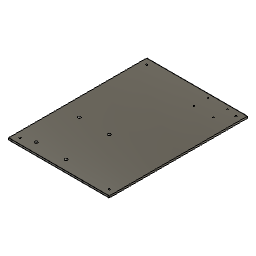
5780 Smaller Board v1 (Autodesk Fusion 360 design; units mm, degrees)
Autodesk Fusion 360 part; units mm, degrees
sketch "Sketch1" plane through (0, 0, 0) normal (0, 0, 1) x (1, 0, 0)
  line L0 (-65, 130) -> (110, 130)
  line L1 (110, 130) -> (110, -110)
  line L2 (110, -110) -> (-65, -110)
  line L3 (-65, -110) -> (-65, 130)
  dimension "d1" = 175
  dimension "d2" = 240
  constraint horizontal L0
  constraint vertical L1
  constraint horizontal L2
  constraint vertical L3
  measures "d1" distance of L1.end L2.end
  measures "d2" distance of L0.start L2.end
extrude "Extrude1" add sketch "Sketch1" along normal blind 3
sketch "Sketch2" plane through (0, 0, 3) normal (0, 0, 1) x (-1, 0, 0)
  line L0 (65, 110) -> (-110, 110)
  line L1 (-110, 110) -> (-110, -130)
  line L2 (-110, -130) -> (65, -130)
  line L3 (65, -130) -> (65, 110)
  circle A0 centre (34.5, 92.5) radius 2.5
  line L4 (60, 5.0001) -> (-105, 5)
  line L5 (12.025, 12.961) -> (3.6107, 13.032) construction
  line L6 (3.6107, 13.032) -> (3.5857, 10.071) construction
  line L7 (3.5857, 10.071) -> (12, 10) construction
  line L8 (12, 10) -> (12.025, 12.961) construction
  line L9 (-105, 5) -> (-105, 105.0001)
  line L10 (-105, 105.0001) -> (60, 105.0001)
  line L11 (12, 100) -> (-4.2428, 100.0343) construction
  line L12 (-4.2428, 100.0343) -> (-4.2609, 91.4763) construction
  line L13 (-4.2609, 91.4763) -> (11.9819, 91.4419) construction
  line L14 (11.9819, 91.4419) -> (12, 100) construction
  line L15 (60, 105.0001) -> (60, 5.0001)
  circle A1 centre (-17.5, 17.5) radius 2.5
  circle A2 centre (-17.5, 92.5) radius 2.5
  circle A3 centre (34.5, 17.5) radius 2.5
  line L16 (-46.15, -125) -> (-84, -125)
  line L17 (-84, -125) -> (-84, -97)
  line L18 (-84, -97) -> (-46.15, -97)
  line L19 (-46.15, -97) -> (-46.15, -125)
  circle A4 centre (-47.975, -123.15) radius 1
  circle A5 centre (-82.175, -123.15) radius 1
  circle A6 centre (-47.975, -98.85) radius 1
  circle A7 centre (-82.175, -98.85) radius 1
  dimension "d33" = 10
  dimension "d34" = 10
  dimension "d7" = 100
  dimension "d8" = 165
  dimension "d9" = 5
  dimension "d10" = 5
  dimension "d11" = 5
  dimension "d12" = 5
  dimension "d13" = 52
  dimension "d14" = 75
  dimension "d15" = 52
  dimension "d16" = 75
  dimension "d17" = 25.5
  dimension "d18" = 25.5
  dimension "d19" = 12.5
  dimension "d20" = 87.5
  dimension "d21" = 12.5
  dimension "d22" = 5
  dimension "d23" = 48
  dimension "d24" = 5
  dimension "d25" = 48
  dimension "d26" = 12.5
  dimension "d27" = 87.5
  dimension "d28" = 5
  dimension "d29" = 5
  dimension "d76" = 37.85
  dimension "d77" = 28
  dimension "d78" = 2
  dimension "d79" = 2
  dimension "d80" = 2
  dimension "d81" = 2
  dimension "d82" = 34.2
  dimension "d83" = 24.3
  dimension "d84" = 34.2
  dimension "d85" = 24.3
  dimension "d86" = 1.825
  dimension "d87" = 1.825
  dimension "d88" = 1.825
  dimension "d89" = 1.825
  dimension "d90" = 1.85
  dimension "d91" = 1.85
  dimension "d92" = 1.85
  dimension "d93" = 1.85
  dimension "d94" = 26
  dimension "d95" = 5
  constraint horizontal L16
  constraint vertical L17
  constraint horizontal L18
  constraint vertical L19
  measures "d7" distance of L4.start L10.end
  measures "d8" distance of L4.start L4.end
  measures "d9" diameter of A3
  measures "d10" diameter of A0
  measures "d11" diameter of A1
  measures "d12" diameter of A2
  measures "d13" distance of A3.centre A1.centre
  measures "d14" distance of A3.centre A0.centre
  measures "d15" distance of A0.centre A2.centre
  measures "d16" distance of A1.centre A2.centre
  measures "d17" distance of A3.centre L15
  measures "d18" distance of A0.centre L15
  measures "d19" distance of A3.centre L4
  measures "d20" distance of A1.centre L9
  measures "d21" distance of A1.centre L4
  measures "d26" distance of A2.centre L10
  measures "d27" distance of A2.centre L9
  measures "d28" distance of L3 L15
  measures "d29" distance of L0 L10
  measures "d76" distance of L16.start L16.end
  measures "d77" distance of L16.start L18.end
  measures "d78" diameter of A4
  measures "d79" diameter of A5
  measures "d80" diameter of A6
  measures "d81" diameter of A7
  measures "d82" distance of A4.centre A5.centre
  measures "d83" distance of A4.centre A6.centre
  measures "d84" horizontal distance of A6.centre A7.centre
  measures "d85" distance of A5.centre A7.centre
  measures "d86" distance of L17 A5.centre
  measures "d87" distance of L17 A7.centre
  measures "d88" distance of L19 A6.centre
  measures "d89" distance of L19 A4.centre
  measures "d90" distance of L16 A4.centre
  measures "d91" distance of L16 A5.centre
  measures "d92" distance of L18 A6.centre
  measures "d93" distance of L18 A7.centre
  measures "d94" distance of L1 L17
  measures "d95" distance of L2 L16
extrude "Extrude2" cut sketch "Sketch2" against normal blind 3 contours A0 | A1 | A2 | A3 | A4 | A5 | A6 | A7
sketch "Sketch3" plane through (0, 0, 3) normal (0, 0, 1) x (-1, 0, 0)
  circle A0 centre (-47.975, -123.15) radius 1
  circle A1 centre (-17.5, 92.5) radius 2.5
  circle A2 centre (34.5, 17.5) radius 2.5
  circle A3 centre (-82.175, -123.15) radius 1
  circle A4 centre (-47.975, -98.85) radius 1
  circle A5 centre (34.5, 92.5) radius 2.5
  circle A6 centre (-17.5, 17.5) radius 2.5
  circle A7 centre (-82.175, -98.85) radius 1
  line L0 (65, 110) -> (-110, 110)
  line L1 (-110, 110) -> (-110, -130)
  line L2 (-110, -130) -> (65, -130)
  line L3 (65, -130) -> (65, 110)
  circle A8 centre (55, -120) radius 1.5
  circle A9 centre (-100, -120) radius 1.5
  circle A10 centre (-100, 100) radius 1.5
  circle A11 centre (55, 100) radius 1.5
  dimension "d98" = 3
  dimension "d99" = 10
  dimension "d100" = 10
  dimension "d101" = 3
  dimension "d102" = 10
  dimension "d103" = 10
  dimension "d104" = 3
  dimension "d105" = 10
  dimension "d106" = 10
  dimension "d107" = 3
  dimension "d108" = 10
  dimension "d109" = 10
  measures "d98" diameter of A8
  measures "d99" distance of L2 A8.centre
  measures "d100" distance of L3 A8.centre
  measures "d101" diameter of A9
  measures "d102" distance of L2 A9.centre
  measures "d103" distance of L1 A9.centre
  measures "d104" diameter of A10
  measures "d105" distance of L0 A10.centre
  measures "d106" distance of L1 A10.centre
  measures "d107" diameter of A11
  measures "d108" distance of L0 A11.centre
  measures "d109" distance of L3 A11.centre
extrude "Extrude3" cut sketch "Sketch3" against normal blind 3 contours A8 | A9 | A10 | A11
